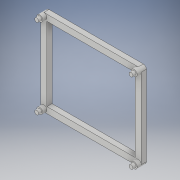
# Autodesk Inventor part: PiMount
Saved by Autodesk Inventor 2018 (Build 220112000, 112)
## iProperties
Created: 2018-01-13
Part Number: PiMount
Material: Generic
Document SubType Name: Modeling
Designer: Kyle-HP
Density: 1 g/cm^3
Appearance: Default
Author: Kyle-HP
Autodesk Inventor part; units mm, degrees
ref_plane "YZ Plane" through (0, 0, 0) normal (1, 0, 0) x (0, 1, 0)
ref_plane "XZ Plane" through (0, 0, 0) normal (0, 1, 0) x (-1, 0, 0)
ref_plane "XY Plane" through (0, 0, 0) normal (0, 0, 1) x (1, 0, 0)
sketch "Sketch1" plane through (0, 0, 0) normal (0, 0, 1) x (1, 0, 0)
  arc A0 (0, 1.905) -> (-1.905, 0) centre (0, 0) ccw
  arc A1 (60.325, 0) -> (58.42, 1.905) centre (58.42, 0) ccw
  arc A2 (-1.905, -49.53) -> (0, -51.435) centre (0, -49.53) ccw
  arc A3 (58.42, -51.435) -> (60.325, -49.53) centre (58.42, -49.53) ccw
  line L0 (0, -51.435) -> (58.42, -51.435)
  line L1 (60.325, -49.53) -> (60.325, 0)
  line L2 (58.42, 1.905) -> (0, 1.905)
  line L3 (-1.905, 0) -> (-1.905, -49.53)
  line L4 (1.905, -47.625) -> (1.905, -1.905)
  line L5 (1.905, -1.905) -> (56.515, -1.905)
  line L6 (56.515, -1.905) -> (56.515, -47.625)
  line L7 (56.515, -47.625) -> (1.905, -47.625)
  dimension "d0" = 58.42
  dimension "d1" = 3.81
  dimension "d2" = 3.81
  dimension "d3" = 49.53
  dimension "d4" = 3.81
  dimension "d5" = 3.81
  constraints: 16 end point, 8 point on circle, 5 coincident, 5 perpendicular, 4 centre point, 2 horizontal, 1 tangent, 1 vertical
  measures "d0" distance of point (58.42, 0) point (0, 0)
  measures "d1" diameter of A0
  measures "d2" diameter of A1
  measures "d3" distance of point (0, -49.53) point (0, 0)
  measures "d4" diameter of A2
  measures "d5" diameter of A3
extrude "Extrusion1" add sketch "Sketch1" along normal blind 3.175
sketch "Sketch2" plane through (0, 0, 3.175) normal (0, 0, 1) x (1, 0, 0)
  circle A0 centre (0, 0) radius 1.2446
  circle A1 centre (58.42, 0) radius 1.2446
  line L0 (60.325, -49.53) -> (60.325, 0) projected
  circle A2 centre (58.42, -49.53) radius 1.2446
  circle A3 centre (0, -49.53) radius 1.2446
  arc A4 (0, 1.905) -> (-1.905, 0) centre (0, 0) ccw projected
  circle A5 centre (0, 0) radius 1.905
  circle A6 centre (0, -49.53) radius 1.905
  circle A7 centre (58.42, -49.53) radius 1.905
  circle A8 centre (58.42, 0) radius 1.905
  dimension "d8" = 2.4892
  dimension "d9" = 2.4892
  dimension "d10" = 1.905
  dimension "d11" = 2.4892
  constraints: 5 centre point, 5 coincident, 3 horizontal alignment, 6 other
  measures "d8" diameter of A0
  measures "d9" diameter of A1
  measures "d10" distance from line of A1.centre L0
  measures "d11" diameter of A2
extrude "Extrusion2" add sketch "Sketch2" along normal blind 4.445 contours A0 | A1 | A2 | A3
extrude "Extrusion3" add sketch "Sketch2" along normal blind 2.54
body "Solid1"
